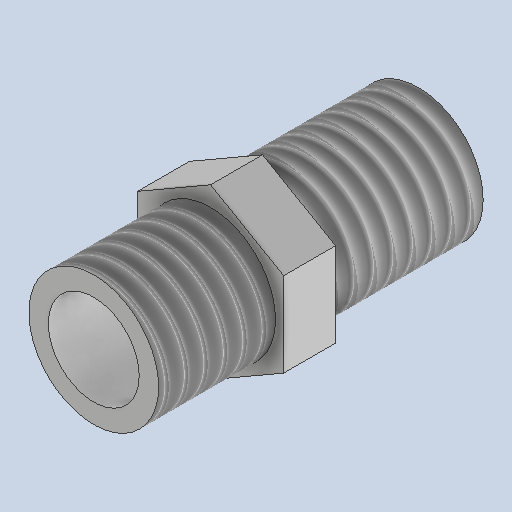
# Autodesk Inventor part: 1154
Saved by Autodesk Inventor 2025.1 (Build 291241000, 241)
## iProperties
Created: 2024-06-07
Part Number: 1154
Material: Generisch
Document SubType Name: Modeling
Designer: ffogue
Density: 1 g/cm^3
Appearance: Vorgabe
Author: ffogue
Autodesk Inventor part; units mm, degrees
ref_plane "YZ Plane" through (0, 0, 0) normal (1, 0, 0) x (0, 1, 0)
ref_plane "XZ Plane" through (0, 0, 0) normal (0, 1, 0) x (-1, 0, 0)
ref_plane "XY Plane" through (0, 0, 0) normal (0, 0, 1) x (1, 0, 0)
sketch "Skizze1" plane through (0, 0, 0) normal (0, 1, 0) x (-1, 0, 0)
  line L0 (0, 6.5) -> (5.6292, 3.25)
  line L1 (5.6292, 3.25) -> (5.6292, -3.25)
  line L2 (5.6292, -3.25) -> (0, -6.5)
  line L3 (0, -6.5) -> (-5.6292, -3.25)
  line L4 (-5.6292, -3.25) -> (-5.6292, 3.25)
  line L5 (-5.6292, 3.25) -> (0, 6.5)
  circle A0 centre (0, 0) radius 5
  dimension "d0" = 10
  dimension "d1" = 13
  constraints: 12 end point, 2 coincident, 1 centre point, 13 other
  measures "d0" diameter of A0
  measures "d1" distance of L2.end L0.start
extrude "Extrusion1" add sketch "Skizze1" along normal mid plane 4
sketch "Skizze2" plane through (0, 2, 0) normal (0, 1, 0) x (1, 0, 0)
  circle A0 centre (0, 0) radius 5
  constraints: 1 centre point, 1 coincident
extrude "Extrusion2" add sketch "Skizze2" along normal blind 12
sketch "Skizze3" plane through (0, 2, 0) normal (0, -1, 0) x (1, 0, 0)
  circle A0 centre (0, 0) radius 5
  constraints: 1 centre point, 1 coincident
extrude "Extrusion3" add sketch "Skizze3" along normal blind 13
thread "Gewinde1" size "M10x1.5" class "6g" standard "ISO Metric profile" length 12
thread "Gewinde2" size "M10x1.5" class "6g" standard "ISO Metric profile" length 9
sketch "Skizze4" plane through (0, 14, 0) normal (0, 1, 0) x (1, 0, 0)
  circle A0 centre (0, 0) radius 3.5
  dimension "d12" = 7
  constraints: 1 centre point, 1 coincident
  measures "d12" diameter of A0
extrude "Extrusion4" cut sketch "Skizze4" against normal up to surface (25 mm away)
